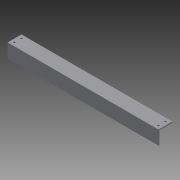
# Autodesk Inventor part: 2x2 angle support
Saved by Autodesk Inventor 2015 SP1 (Build 190203100, 203)
## iProperties
Created: 2015-01-17
Part Number: 2x2 angle support
Material: Generic
Document SubType Name: Modeling
Designer: Jarod
Density: 1 g/cm^3
Appearance: Default
Author: Jarod
Autodesk Inventor part; units mm, degrees
ref_plane "YZ Plane" through (0, 0, 0) normal (1, 0, 0) x (0, 1, 0)
ref_plane "XZ Plane" through (0, 0, 0) normal (0, 1, 0) x (-1, 0, 0)
ref_plane "XY Plane" through (0, 0, 0) normal (0, 0, 1) x (1, 0, 0)
sketch "Sketch1" plane through (0, 0, 0) normal (1, 0, 0) x (0, 1, 0)
  line L0 (0, 0) -> (-50.8, 0)
  line L1 (-50.8, 0) -> (-50.8, -3.175)
  line L2 (-50.8, -3.175) -> (0, -3.175)
  line L3 (0, -3.175) -> (0, 0)
  line L4 (0, 0) -> (-3.175, 0)
  line L5 (-3.175, 0) -> (-3.175, -50.8)
  line L6 (-3.175, -50.8) -> (0, -50.8)
  line L7 (0, -50.8) -> (0, 0)
  dimension "d0" = 50.8
  dimension "d1" = 3.175
  dimension "d2" = 3.175
  dimension "d3" = 50.8
  constraints: 16 end point, 4 parallel, 2 horizontal, 2 perpendicular
  measures "d0" distance of L2.end L1.end
  measures "d1" distance of L1.end L0.end
  measures "d2" distance of L6.end L5.end
  measures "d3" distance of L5.end L4.end
extrude "Extrusion1" add sketch "Sketch1" along normal blind 552.45
sketch "Sketch2" plane through (0, 0, 0) normal (0, 1, 0) x (1, 0, 0)
  line L0 (0, 50.8) -> (0, 0) projected
  line L1 (0, 0) -> (552.45, 0) projected
  line L2 (552.45, 50.8) -> (552.45, 0) projected
  line L3 (0, 50.8) -> (552.45, 50.8) projected
  point P0 (12.7, 12.7)
  point P1 (12.7, 38.1)
  point P2 (539.75, 12.7)
  point P3 (539.75, 38.1)
  dimension "d6" = 12.7
  dimension "d7" = 12.7
  dimension "d8" = 12.7
  dimension "d9" = 12.7
  dimension "d10" = 12.7
  dimension "d11" = 12.7
  dimension "d12" = 12.7
  dimension "d13" = 12.7
  measures "d6" distance from line of L1 point (539.75, 12.7)
  measures "d7" distance from line of L2 point (539.75, 12.7)
  measures "d8" distance from line of L3 point (539.75, 38.1)
  measures "d9" distance from line of L2 point (539.75, 38.1)
  measures "d10" distance from line of L0 point (12.7, 12.7)
  measures "d11" distance from line of L1 point (12.7, 12.7)
  measures "d12" distance from line of L0 point (12.7, 38.1)
  measures "d13" distance from line of L3 point (12.7, 38.1)
hole "Hole1" at (12.7, 0, -12.7) at (12.7, 0, -38.1) at (539.75, 0, -12.7) at (539.75, 0, -38.1) direction (0, -1, 0) diameter 6.35 end through all
body "Solid1"
